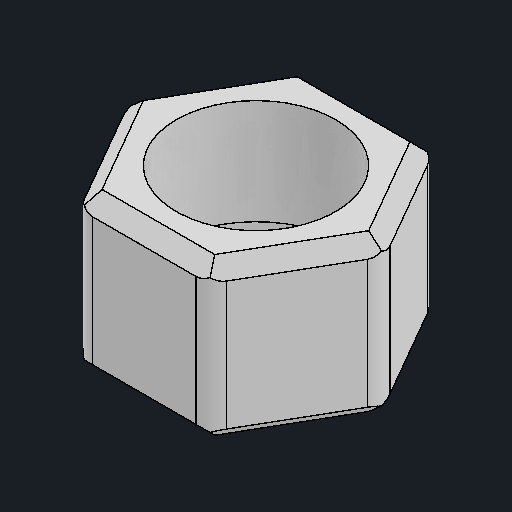
# Autodesk Inventor part: 40mm Nut
Saved by Autodesk Inventor 2026.2 (Build 302298000, 298)
## iProperties
Created: 2026-06-22
Part Number: 40mm Nut
Material: Generic
Document SubType Name: Modeling
Designer: Joshua Eah
Density: 1 g/cm^3
Appearance: Default
Author: Joshua Eah
Autodesk Inventor part; units mm, degrees
ref_plane "YZ Plane" through (0, 0, 0) normal (1, 0, 0) x (0, 1, 0)
ref_plane "XZ Plane" through (0, 0, 0) normal (0, 1, 0) x (-1, 0, 0)
ref_plane "XY Plane" through (0, 0, 0) normal (0, 0, 1) x (1, 0, 0)
sketch "Sketch1" plane through (0, 0, 0) normal (0, 1, 0) x (-1, 0, 0)
  circle A0 centre (0, 0) radius 20
  circle A1 centre (0, 0) radius 25
  line L0 (-14.4338, -25) -> (-28.8675, 0)
  line L1 (-28.8675, 0) -> (-14.4338, 25)
  line L2 (-14.4338, 25) -> (14.4338, 25)
  line L3 (14.4338, 25) -> (28.8675, 0)
  line L4 (28.8675, 0) -> (14.4338, -25)
  line L5 (14.4338, -25) -> (-14.4338, -25)
  point P0 (0, -25)
  point P1 (21.6506, -12.5)
  point P2 (-21.6506, -12.5)
  point P3 (21.6506, 12.5)
  point P4 (0, 25)
  point P5 (-21.6506, 12.5)
  dimension "d0" = 40
  dimension "d1" = 50
  constraints: 12 end point, 2 centre point, 2 coincident, 1 concentric, 1 horizontal, 1 tangent, 13 other
  measures "d0" diameter of A0
  measures "d1" diameter of A1
extrude "Extrusion1" add sketch "Sketch1" against normal blind 10
extrude "Extrusion2" add sketch "Sketch1" along normal blind 25 separate body
draft "FaceDraft1" angle 5 pull direction (0, -1, 0) faces at (-19.9351, 16.6667, -1.6093) fixed edges at (20, 0, 0) (20, 0, 0)
combine bodies "Combine1" operation type add bodies to combine 1 2
chamfer "Chamfer1" distance 3.175 angle 45 12 edges at (0, 25, 25) (21.6506, 25, 12.5) (21.6506, 25, -12.5) (0, 25, -25) (-21.6506, 25, -12.5) (-21.6506, 25, 12.5) (0, -10, 25) (-21.6506, -10, 12.5) (21.6506, -10, 12.5) (21.6506, -10, -12.5) (0, -10, -25) (-21.6506, -10, -12.5)
fillet "Fillet1" radius 5 6 edges at (-14.4338, 7.5, -25) (-28.8675, 7.5, 0) (14.4338, 7.5, -25) (28.8675, 7.5, 0) (14.4338, 7.5, 25) (-14.4338, 7.5, 25)
body "Solid1"
